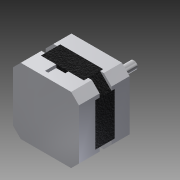
# Autodesk Inventor part: NEMA17
Saved by Autodesk Inventor 2015 (Build 190159000, 159)
## iProperties
Created: 2015-04-13
Part Number: NEMA17
Material: Generic
Document SubType Name: Modeling
Designer: IEUser
Density: 1 g/cm^3
Appearance: Default
Author: IEUser
Autodesk Inventor part; units mm, degrees
ref_plane "YZ Plane" through (0, 0, 0) normal (1, 0, 0) x (0, 1, 0)
ref_plane "XZ Plane" through (0, 0, 0) normal (0, 1, 0) x (-1, 0, 0)
ref_plane "XY Plane" through (0, 0, 0) normal (0, 0, 1) x (1, 0, 0)
sketch "captive_nut_mortises" plane through (0, 0, 0) normal (0, 0, 1) x (1, 0, 0)
  circle A0 centre (0, 0) radius 1.5
  line L0 (14, -2) -> (10, -2)
  line L1 (10, -2) -> (10, 2)
  line L2 (10, 2) -> (14, 2)
  line L3 (14, 2) -> (14, -2)
  line L4 (-10, -2) -> (-14, -2)
  line L5 (-14, -2) -> (-14, 2)
  line L6 (-14, 2) -> (-10, 2)
  line L7 (-10, 2) -> (-10, -2)
  line L8 (10, 0) -> (-10, 0) construction
  dimension "SCREW_HOLE_SIZE" = 3
  dimension "MORTISE_LENGTH" = 4
  dimension "MORTISE_WIDTH" = 4
  dimension "MORTISES_INTERVAL" = 20
  measures "SCREW_HOLE_SIZE" diameter of A0
  measures "MORTISE_LENGTH" distance of L1.end L2.end
  measures "MORTISE_WIDTH" distance of L2.end L0.start
  measures "MORTISES_INTERVAL" distance of L8.start L8.end
sketch "captive_nut_tenons" plane through (0, 0, 0) normal (0, 0, 1) x (1, 0, 0)
  line L0 (-13.7959, 1.2254) -> (-9.7959, 1.2254)
  line L1 (-9.7959, 1.2254) -> (-9.7959, -2.7746)
  line L2 (-13.7959, -2.7746) -> (-13.7959, 1.2254)
  line L3 (10.2041, 1.2254) -> (14.2041, 1.2254)
  line L4 (14.2041, 1.2254) -> (14.2041, -2.7746)
  line L5 (10.2041, -2.7746) -> (10.2041, 1.2254)
  line L6 (-1.2959, -2.7746) -> (-1.2959, -10.2746)
  line L7 (-1.2959, -10.2746) -> (-2.7959, -10.2746)
  line L8 (-2.7959, -10.2746) -> (-2.7959, -13.2746)
  line L9 (-2.7959, -13.2746) -> (-1.2959, -13.2746)
  line L10 (-1.2959, -13.2746) -> (-1.2959, -14.7746)
  line L11 (-1.2959, -14.7746) -> (1.7041, -14.7746)
  line L12 (1.7041, -14.7746) -> (1.7041, -13.2746)
  line L13 (1.7041, -13.2746) -> (3.2041, -13.2746)
  line L14 (3.2041, -13.2746) -> (3.2041, -10.2746)
  line L15 (3.2041, -10.2746) -> (1.7041, -10.2746)
  line L16 (1.7041, -2.7746) -> (1.7041, -10.2746)
  line L17 (-9.7959, -2.7746) -> (-1.2959, -2.7746)
  line L18 (1.7041, -2.7746) -> (10.2041, -2.7746)
  point P0 (3.4972, 2.1027)
  dimension "TENONS_INTERVAL" = 20
  dimension "TENON_LENGTH" = 4
  dimension "TENON_WIDTH" = 4
  dimension "SCREW_SIZE" = 3
  dimension "SCREW_LENGTH" = 12
  dimension "NUT_THICKNESS" = 3
  dimension "NUT_DEPTH" = 7.5
  dimension "NUT_WIDTH" = 6
  measures "TENONS_INTERVAL" distance of L1.end L5.start
  measures "TENON_LENGTH" distance of L3.end L4.end
  measures "TENON_WIDTH" distance of L3.start L3.end
  measures "SCREW_SIZE" distance of L10.end L11.end
  measures "SCREW_LENGTH" distance of L16.start L11.end
  measures "NUT_THICKNESS" distance of L13.end L14.end
  measures "NUT_DEPTH" distance of L16.start L15.end
  measures "NUT_WIDTH" distance of L13.end L8.end
sketch "Sketch3" plane through (0, 0, 0) normal (0, 1, 0) x (-1, 0, 0)
  line L0 (16.15, 21.15) -> (-16.15, 21.15)
  line L1 (-21.15, 16.15) -> (-21.15, -16.15)
  line L2 (-16.15, -21.15) -> (16.15, -21.15)
  line L3 (21.15, -16.15) -> (21.15, 16.15)
  line L4 (26.9622, 0) -> (-36.6505, 0) construction
  line L5 (0, 25.1398) -> (0, -25.5601) construction
  line L6 (16.15, 21.15) -> (21.15, 16.15)
  line L7 (-21.15, -16.15) -> (-16.15, -21.15)
  line L8 (16.15, -21.15) -> (21.15, -16.15)
  line L9 (-16.15, 21.15) -> (-21.15, 16.15)
  point P0 (0, 0)
  point P1 (21.15, 21.15)
  point P2 (-21.15, -21.15)
  point P3 (-21.15, 21.15)
  point P4 (21.15, -21.15)
  point P5 (0, 0)
  dimension "d13" = 42.3
  dimension "d14" = 42.3
  dimension "d15" = 5
  dimension "d16" = 5
  dimension "d17" = 5
  dimension "d18" = 5
  dimension "d19" = 5
  dimension "d20" = 5
  dimension "d21" = 5
  dimension "d22" = 5
  constraints: 20 end point, 8 point on line, 2 horizontal, 2 parallel, 1 perpendicular, 1 vertical
  measures "d13" distance of point (21.15, -21.15) point (21.15, 21.15)
  measures "d14" distance of point (21.15, 21.15) point (-21.15, 21.15)
  measures "d15" distance of L0.start point (21.15, 21.15)
  measures "d16" distance of L3.end point (21.15, 21.15)
  measures "d17" distance of L1.end point (-21.15, -21.15)
  measures "d18" distance of L2.start point (-21.15, -21.15)
  measures "d19" distance of L2.end point (21.15, -21.15)
  measures "d20" distance of L3.start point (21.15, -21.15)
  measures "d21" distance of L0.end point (-21.15, 21.15)
  measures "d22" distance of L1.start point (-21.15, 21.15)
extrude "Extrusion1" add sketch "Sketch3" along normal blind 10.5
sketch "Sketch5" plane through (0, 10.5, 0) normal (0, 1, 0) x (1, 0, 0)
  line L0 (-21.15, -16.15) -> (-16.15, -21.15)
  line L1 (-21.15, -16.15) -> (-16.15, -21.15) projected
  line L2 (-16.15, -21.15) -> (-13.7, -21.15)
  line L3 (-13.7, -21.15) -> (-21.15, -13.7)
  line L4 (-21.15, -13.7) -> (-21.15, -16.15)
  line L5 (16.15, -21.15) -> (21.15, -16.15)
  line L6 (21.15, -16.15) -> (21.15, -13.7)
  line L7 (21.15, -13.7) -> (13.7, -21.15)
  line L8 (13.7, -21.15) -> (16.15, -21.15)
  line L9 (21.15, 16.15) -> (16.15, 21.15)
  line L10 (16.15, 21.15) -> (13.7, 21.15)
  line L11 (13.7, 21.15) -> (21.15, 13.7)
  line L12 (21.15, 13.7) -> (21.15, 16.15)
  line L13 (-16.15, 21.15) -> (-21.15, 16.15)
  line L14 (-21.15, 16.15) -> (-21.15, 13.7)
  line L15 (-21.15, 13.7) -> (-13.7, 21.15)
  line L16 (-13.7, 21.15) -> (-16.15, 21.15)
  point P0 (0, 0)
  dimension "d29" = 2.45
  dimension "d30" = 2.45
  dimension "d33" = 360
  constraints: 32 end point, 1 collinear, 1 parallel, 1 perpendicular, 33 other
  measures "d29" distance of L3.end L0.start
  measures "d30" distance of L0.end L2.end
extrude "Extrusion2" add sketch "Sketch5" along normal blind 2.8
sketch "Sketch6" plane through (0, 10.5, 0) normal (0, 1, 0) x (1, 0, 0)
  line L0 (21.15, 13.7) -> (13.7, 21.15) projected
  line L1 (13.7, 21.15) -> (-13.7, 21.15) projected
  line L2 (-13.7, 21.15) -> (-21.15, 13.7) projected
  line L3 (-21.15, 13.7) -> (-21.15, -13.7) projected
  line L4 (-21.15, -13.7) -> (-13.7, -21.15) projected
  line L5 (-13.7, -21.15) -> (13.7, -21.15) projected
  line L6 (13.7, -21.15) -> (21.15, -13.7) projected
  line L7 (21.15, -13.7) -> (21.15, 13.7) projected
  point P0 (0, 0)
extrude "Extrusion3" add sketch "Sketch6" along normal blind 12.4 separate body
sketch "Sketch7" plane through (0, 22.9, 0) normal (0, 1, 0) x (1, 0, 0)
  line L0 (16.15, -21.15) -> (21.15, -16.15) projected
  line L1 (13.7, -21.15) -> (16.15, -21.15) projected
  line L2 (-13.7, -21.15) -> (13.7, -21.15) projected
  line L3 (-16.15, -21.15) -> (-13.7, -21.15) projected
  line L4 (-21.15, -16.15) -> (-16.15, -21.15) projected
  line L5 (-21.15, -13.7) -> (-21.15, -16.15) projected
  line L6 (-21.15, 13.7) -> (-21.15, -13.7) projected
  line L7 (-21.15, 16.15) -> (-21.15, 13.7) projected
  line L8 (-16.15, 21.15) -> (-21.15, 16.15) projected
  line L9 (13.7, 21.15) -> (-13.7, 21.15) projected
  line L10 (-13.7, 21.15) -> (-16.15, 21.15) projected
  line L11 (16.15, 21.15) -> (13.7, 21.15) projected
  line L12 (21.15, 16.15) -> (16.15, 21.15) projected
  line L13 (21.15, -13.7) -> (21.15, 13.7) projected
  line L14 (21.15, 13.7) -> (21.15, 16.15) projected
  line L15 (21.15, -16.15) -> (21.15, -13.7) projected
  point P0 (0, 0)
extrude "Extrusion4" add sketch "Sketch7" along normal blind 9.6 separate body
sketch "Sketch8" plane through (0, 22.9, 0) normal (0, -1, 0) x (1, 0, 0)
  line L0 (16.15, 21.15) -> (21.15, 16.15) projected
  line L1 (21.15, 16.15) -> (21.15, 13.7) projected
  line L2 (21.15, 13.7) -> (13.7, 21.15) projected
  line L3 (13.7, 21.15) -> (16.15, 21.15) projected
  line L4 (-21.15, 16.15) -> (-16.15, 21.15) projected
  line L5 (-16.15, 21.15) -> (-13.7, 21.15) projected
  line L6 (-13.7, 21.15) -> (-21.15, 13.7) projected
  line L7 (-21.15, 13.7) -> (-21.15, 16.15) projected
  line L8 (-16.15, -21.15) -> (-21.15, -16.15) projected
  line L9 (-21.15, -16.15) -> (-21.15, -13.7) projected
  line L10 (-21.15, -13.7) -> (-13.7, -21.15) projected
  line L11 (-13.7, -21.15) -> (-16.15, -21.15) projected
  line L12 (21.15, -16.15) -> (16.15, -21.15) projected
  line L13 (16.15, -21.15) -> (13.7, -21.15) projected
  line L14 (13.7, -21.15) -> (21.15, -13.7) projected
  line L15 (21.15, -13.7) -> (21.15, -16.15) projected
  point P0 (0, 0)
extrude "Extrusion5" add sketch "Sketch8" along normal blind 2 bodies 3
sketch "Sketch9" plane through (-16.15, 0, 21.15) normal (0, 0, 1) x (1, 0, 0)
  line L0 (32.3, 0) -> (0, 0) projected
  line L1 (12.25, 10.5) -> (20.05, 10.5)
  line L2 (20.05, 10.5) -> (20.05, 3.3)
  line L3 (20.05, 3.3) -> (12.25, 3.3)
  line L4 (12.25, 3.3) -> (12.25, 10.5)
  line L5 (2.45, 10.5) -> (29.85, 10.5) projected
  point P0 (16.15, 0)
  dimension "d43" = 7.8
  dimension "d44" = 3.9
  dimension "d45" = 7.2
  constraints: 8 end point, 2 parallel, 1 collinear, 1 horizontal, 1 perpendicular
  measures "d43" distance between parallel lines of L2 L4
  measures "d44" distance from line of point (16.15, 0) L4
  measures "d45" distance of L3.end L1.start
extrude "Extrusion6" cut sketch "Sketch9" against normal blind 2 bodies 1
sketch "Sketch10" plane through (0, 32.5, 0) normal (0, 1, 0) x (1, 0, 0)
  circle A0 centre (15.5, 15.5) radius 1
  circle A1 centre (-15.5, 15.5) radius 1
  circle A2 centre (-15.5, -15.5) radius 1
  circle A3 centre (15.5, -15.5) radius 1
  point P0 (0, 0)
  dimension "d48" = 2
  dimension "d49" = 15.5
  dimension "d50" = 15.5
  dimension "d53" = 360
  constraints: 4 centre point, 9 other
  measures "d48" diameter of A0
  measures "d49" horizontal distance of point (0, 0) A0.centre
  measures "d50" horizontal distance of point (0, 0) A0.centre
extrude "Extrusion7" cut sketch "Sketch10" against normal blind 4 bodies 3
sketch "Sketch11" plane through (0, 32.5, 0) normal (0, 1, 0) x (1, 0, 0)
  circle A0 centre (0, 0) radius 11
  dimension "d57" = 22
  constraints: 1 centre point, 1 coincident
  measures "d57" diameter of A0
extrude "Extrusion8" add sketch "Sketch11" along normal blind 2 bodies 3
sketch "Sketch12" plane through (0, 34.5, 0) normal (0, 1, 0) x (1, 0, 0)
  circle A0 centre (0, 0) radius 5.8653
  constraints: 1 centre point, 1 coincident
extrude "Extrusion9" cut sketch "Sketch12" against normal blind 3 bodies 3
sketch "Sketch13" plane through (0, 31.5, 0) normal (0, 1, 0) x (1, 0, 0)
  circle A0 centre (0, 0) radius 2.5
  dimension "d62" = 5
  constraints: 1 centre point, 1 coincident
  measures "d62" diameter of A0
extrude "Extrusion10" add sketch "Sketch13" along normal blind 25 separate body
chamfer "Chamfer1" distance 0.25 angle 45 1 edges at (-2.5, 56.5, 0)
sketch "Sketch14" plane through (0, 56.5, 0) normal (0, 1, 0) x (1, 0, 0)
  circle A0 centre (0, 0) radius 1
  dimension "d68" = 2
  constraints: 1 centre point, 1 coincident
  measures "d68" diameter of A0
extrude "Extrusion11" cut sketch "Sketch14" against normal blind 2 bodies 4
equation "\"d16\" = d15"
equation "\"d17\" = d15"
equation "\"d18\" = d17"
equation "\"d19\" = d15"
equation "\"d20\" = d19"
equation "\"d21\" = d15"
equation "\"d22\" = d21"
equation "\"d50\" = d49"
equation "\"NUT_DEPTH\" = SCREW_LENGTH - 1.5 * NUT_THICKNESS"
